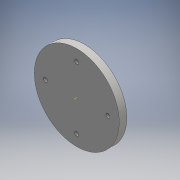
# Autodesk Inventor part: Motor Mount Barebones bigscrew4mmheight
Saved by Autodesk Inventor 2016 SP1 (Build 200210100, 210)
## iProperties
Created: 2017-05-01
Part Number: Motor Mount Barebones bigscrew4mmheight
Material: Generic
Document SubType Name: Modeling
Designer: mundhend06
Density: 1 g/cm^3
Appearance: Default
Author: mundhend06
Autodesk Inventor part; units mm, degrees
ref_plane "YZ Plane" through (0, 0, 0) normal (1, 0, 0) x (0, 1, 0)
ref_plane "XZ Plane" through (0, 0, 0) normal (0, 1, 0) x (-1, 0, 0)
ref_plane "XY Plane" through (0, 0, 0) normal (0, 0, 1) x (1, 0, 0)
sketch "Sketch1" plane through (0, 0, 0) normal (0, 1, 0) x (-1, 0, 0)
  circle A0 centre (0, 0) radius 22.5
  dimension "d0" = 45
  constraints: 1 centre point, 1 coincident
  measures "d0" diameter of A0
extrude "Extrusion1" add sketch "Sketch1" along normal blind 4
sketch "Sketch2" plane through (0, 4, 0) normal (0, 1, 0) x (1, 0, 0)
  line L0 (0, 0) -> (0, 8) construction
  line L1 (0, 0) -> (0, -8) construction
  circle A0 centre (0, 8) radius 1.9
  circle A1 centre (0, 0) radius 1.9
  circle A2 centre (0, -8) radius 1.9
  dimension "d3" = 8
  dimension "d4" = 8
  dimension "d5" = 3.8
  dimension "d6" = 3.8
  dimension "d7" = 3.8
  constraints: 4 end point, 3 centre point, 3 coincident, 2 vertical
  measures "d3" distance of L0.start L0.end
  measures "d4" distance of L0.start L1.end
  measures "d5" diameter of A0
  measures "d6" diameter of A1
  measures "d7" diameter of A2
extrude "Extrusion2" add sketch "Sketch2" along normal blind 10
sketch "Sketch7" plane through (0, 0, 0) normal (0, -1, 0) x (1, 0, 0)
  circle A0 centre (0, 0) radius 16.5 construction
  circle A1 centre (0, 16.5) radius 1.05
  circle A2 centre (16.5, 0) radius 1.05
  circle A3 centre (-16.5, 0) radius 1.05
  circle A4 centre (0, -16.5) radius 1.05
  dimension "d42" = 33
  dimension "d43" = 2.1
  dimension "d44" = 2.1
  dimension "d45" = 2.1
  dimension "d46" = 2.1
  constraints: 5 centre point, 4 point on circle, 1 coincident
  measures "d42" diameter of A0
  measures "d43" diameter of A1
  measures "d44" diameter of A2
  measures "d45" diameter of A3
  measures "d46" diameter of A4
extrude "Extrusion6" cut sketch "Sketch7" against normal blind 5
body "Solid1"
